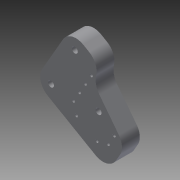
# Autodesk Inventor part: joint3+ax12imprint_v2
Saved by Autodesk Inventor 2014 (Build 180170000, 170)
## iProperties
Created: 2014-01-12
Part Number: joint3+ax12imprint_v2
Material: Générique
Document SubType Name: Modeling
Designer: helly
Density: 1 g/cm^3
Appearance: Par défaut
Author: helly
Autodesk Inventor part; units mm, degrees
ref_plane "YZ Plane" through (0, 0, 0) normal (1, 0, 0) x (0, 1, 0)
ref_plane "XZ Plane" through (0, 0, 0) normal (0, 1, 0) x (-1, 0, 0)
ref_plane "XY Plane" through (0, 0, 0) normal (0, 0, 1) x (1, 0, 0)
sketch "Esquisse1" plane through (0, 0, 0) normal (0, 1, 0) x (-1, 0, 0)
  line L0 (0, 0) -> (32, 0) construction
  line L1 (32, 0) -> (16, 27.7128) construction
  line L2 (16, 27.7128) -> (0, 0) construction
  line L3 (-10.3913, 17.9982) -> (9.0252, -15.6322) construction
  line L4 (8, -13.8564) -> (32, 0) construction
  line L5 (8, -13.8564) -> (14.9282, -9.8564) construction
  line L6 (8, -13.8564) -> (-10, 17.3205) construction
  line L7 (-10, 17.3205) -> (1.6913, 24.0705) construction
  line L8 (1.6913, 24.0705) -> (4.9413, 18.4413) construction
  line L9 (4.9413, 18.4413) -> (8.9413, 11.5131) construction
  line L10 (8.9413, 11.5131) -> (12.9413, 4.5849) construction
  line L11 (12.9413, 4.5849) -> (16.9413, -2.3433) construction
  circle A0 centre (8.9413, 11.5131) radius 1
  circle A1 centre (12.9413, 4.5849) radius 1
  circle A2 centre (16.9413, -2.3433) radius 1
  circle A3 centre (14.9282, -9.8564) radius 1
  circle A4 centre (4.9413, 18.4413) radius 1
  circle A5 centre (-14.4413, -1.9869) radius 1 construction
  circle A6 centre (-10.4413, -8.9151) radius 1
  circle A7 centre (-6.4413, -15.8433) radius 1
  circle A8 centre (1.0718, -17.8564) radius 1
  circle A9 centre (-18.4413, 4.9413) radius 1 construction
  circle A10 centre (-10, 17.3205) radius 11.6 construction
  line L12 (32, 0) -> (36, -6.9282) construction
  line L13 (36.0415, 0) -> (34.0207, -3.5) construction
  line L14 (34.0207, -3.5) -> (29.9793, -3.5) construction
  line L15 (29.9793, -3.5) -> (27.9585, 0) construction
  line L16 (27.9585, 0) -> (29.9793, 3.5) construction
  line L17 (29.9793, 3.5) -> (34.0207, 3.5) construction
  line L18 (34.0207, 3.5) -> (36.0415, 0) construction
  line L19 (34.0207, 3.5) -> (34.0207, -3.5) construction
  circle A11 centre (16, 27.7128) radius 2
  circle A12 centre (32, 0) radius 2
  line L20 (32, 0) -> (38.9282, 4) construction
  line L21 (-6.4413, -15.8433) -> (-13.3695, -19.8433) construction
  line L22 (42.9282, -2.9282) -> (-6.6195, -31.5346)
  line L23 (-6.6195, -31.5346) -> (-30.6195, 10.0346)
  line L24 (-30.6195, 10.0346) -> (18.9282, 38.641)
  line L25 (18.9282, 38.641) -> (42.9282, -2.9282)
  line L26 (8, -13.8564) -> (12, -20.7846) construction
  line L27 (16, 27.7128) -> (12, 34.641) construction
  circle A13 centre (0, 0) radius 2
  dimension "d0" = 32
  dimension "d1" = 32
  dimension "d2" = 60
  dimension "d4" = 8
  dimension "d6" = 36
  dimension "d7" = 13.5
  dimension "d8" = 6.5
  dimension "d9" = 8
  dimension "d10" = 8
  dimension "d11" = 8
  dimension "d13" = 2
  dimension "d14" = 11.6
  dimension "d15" = 8
  dimension "d16" = 7
  dimension "d17" = 4
  dimension "d19" = 8
  dimension "d20" = 8
  dimension "d26" = 8
  dimension "d27" = 8
  constraints: 56 end point, 14 centre point, 11 coincident, 11 point on line, 8 perpendicular, 6 equal radius, 5 collinear, 5 symmetric about line, 4 parallel, 1 horizontal, 18 other
  measures "d0" distance of L0.start L0.end
  measures "d1" distance of L0.end L1.end
  measures "d2" angle of L1 L0
  measures "d4" distance of L4.start L5.end
  measures "d6" distance of L4.start L6.end
  measures "d7" distance of L6.end L7.end
  measures "d8" distance of L7.end L8.end
  measures "d9" distance of L8.end L9.end
  measures "d10" distance of L9.end L10.end
  measures "d11" distance of L10.end L11.end
  measures "d13" diameter of A4
  measures "d14" radius of A10
  measures "d15" distance of L4.end L12.end
  measures "d16" distance of L17.end L13.end
  measures "d17" diameter of A11
  measures "d19" distance of L20.start L20.end
  measures "d20" distance of L21.start L21.end
  measures "d26" distance of L4.start L26.end
  measures "d27" distance of L27.start L27.end
extrude "Extrusion4" add sketch "Esquisse1" along normal blind 12
sketch "Esquisse7" plane through (0, 12, 0) normal (0, 1, 0) x (1, 0, 0)
  circle A0 centre (10.4413, 8.9151) radius 1 projected
  circle A1 centre (-4.9413, -18.4413) radius 1 projected
  line L0 (-18.9282, -38.641) -> (30.6195, -10.0346) projected
  line L1 (30.6195, -10.0346) -> (6.6195, 31.5346) projected
  line L2 (-4.9413, -18.4413) -> (-1.6913, -24.0705) construction
  line L3 (-1.6913, -24.0705) -> (10, -17.3205) construction
  circle A2 centre (10, -17.3205) radius 12 construction
  line L4 (10.4413, 8.9151) -> (12.4413, 5.451) construction
  line L5 (-0.3923, -23.3205) -> (1.6077, -26.7846)
  line L6 (17.7305, 12.2898) -> (0.5077, -9.9791)
  arc A3 (0.5077, -9.9791) -> (-0.3923, -23.3205) centre (10, -17.3205) ccw
  dimension "d54" = 6.5
  dimension "d55" = 13.5
  dimension "d56" = 24
  dimension "d57" = 4
  constraints: 10 end point, 4 point on circle, 4 point on line, 3 perpendicular, 2 centre point, 2 coincident, 1 parallel, 1 tangent
  measures "d54" distance of L2.start L2.end
  measures "d55" distance of L2.end L3.end
  measures "d56" diameter of A2
  measures "d57" distance of L4.start L4.end
extrude "Extrusion5" cut sketch "Esquisse7" against normal through all contours L5 A3 L6 L1 L0
fillet "Congé8" radius 10 1 edges at (1.6077, 6, 26.7846)
fillet "Congé9" radius 10 1 edges at (17.7305, 6, -12.2898)
fillet "Congé10" radius 10 1 edges at (6.6195, 6, -31.5346)
fillet "Congé11" radius 10 1 edges at (-42.9282, 6, -2.9282)
fillet "Congé12" radius 10 1 edges at (-18.9282, 6, 38.641)
sketch "Esquisse8" plane through (0, 12, 0) normal (0, 1, 0) x (1, 0, 0)
  circle A0 centre (0, 0) radius 2 projected
  circle A1 centre (-32, 0) radius 2 projected
  circle A2 centre (-16, -27.7128) radius 2 projected
  circle A3 centre (6.4413, 15.8433) radius 1 projected
  circle A4 centre (10.4413, 8.9151) radius 1 projected
  line L0 (-2.0407, 26.5346) -> (-34.2679, 7.9282) projected
  line L1 (-28.5, 2.0207) -> (-28.5, -2.0207)
  line L2 (-28.5, -2.0207) -> (-32, -4.0415)
  line L3 (-32, -4.0415) -> (-35.5, -2.0207)
  line L4 (-35.5, -2.0207) -> (-35.5, 2.0207)
  line L5 (-35.5, 2.0207) -> (-32, 4.0415)
  line L6 (-32, 4.0415) -> (-28.5, 2.0207)
  line L7 (-19.5, -25.6921) -> (-16, -23.6714)
  line L8 (-16, -23.6714) -> (-12.5, -25.6921)
  line L9 (-12.5, -25.6921) -> (-12.5, -29.7335)
  line L10 (-12.5, -29.7335) -> (-16, -31.7543)
  line L11 (-16, -31.7543) -> (-19.5, -29.7335)
  line L12 (-19.5, -29.7335) -> (-19.5, -25.6921)
  line L13 (-32, 4.0415) -> (-28.5, -2.0207) construction
  line L14 (0, 4.0415) -> (3.5, 2.0207)
  line L15 (3.5, 2.0207) -> (3.5, -2.0207)
  line L16 (3.5, -2.0207) -> (0, -4.0415)
  line L17 (0, -4.0415) -> (-3.5, -2.0207)
  line L18 (-3.5, -2.0207) -> (-3.5, 2.0207)
  line L19 (-3.5, 2.0207) -> (0, 4.0415)
  dimension "d66" = 7
  constraints: 38 end point, 5 coincident, 3 parallel, 2 equal length, 39 other
  measures "d66" distance of L1.end L5.end
extrude "Extrusion6" cut sketch "Esquisse8" against normal blind 3 contours L1 L2 L3 L4 L5 L6 | L7 L8 L9 L10 L11 L12 | L14 L15 L16 L17 L18 L19
